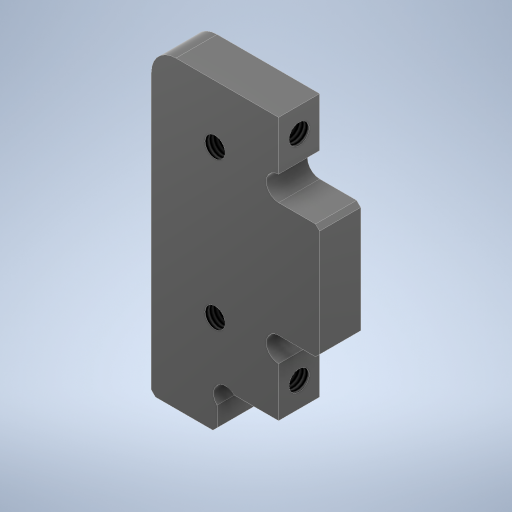
# Autodesk Inventor part: TorsoAngleBraceFrame
Saved by Autodesk Inventor 2024.2 (Build 282272000, 272)
## iProperties
Created: 2024-01-21
Part Number: TorsoAngleBraceFrame
Material: Acetal Resin, Black
Document SubType Name: Modeling
Designer: Masato Kubotera
Density: 1.425 g/cm^3
Appearance: Smooth - Black
Mass: 4.09203 g
Surface Area: 19.2357 cm^2
Volume: 2.8716 cm^3
Vendor: meviy
Author: Masato Kubotera
Autodesk Inventor part; units mm, degrees
ref_plane "YZ Plane" through (0, 0, 0) normal (1, 0, 0) x (0, 1, 0)
ref_plane "XZ Plane" through (0, 0, 0) normal (0, 1, 0) x (-1, 0, 0)
ref_plane "XY Plane" through (0, 0, 0) normal (0, 0, 1) x (1, 0, 0)
sketch "Sketch1" plane through (0, 0, 0) normal (1, 0, 0) x (0, 1, 0)
  line L0 (0.25, 0) -> (0.25, -5)
  line L1 (0.25, -5) -> (-7.75, -5)
  line L2 (-7.75, -5) -> (-7.75, 32)
  line L3 (-7.75, 32) -> (7.75, 32)
  line L4 (7.75, 32) -> (7.75, 23)
  line L5 (7.75, 23) -> (12.75, 23)
  line L6 (12.75, 23) -> (12.75, 9)
  line L7 (12.75, 9) -> (7.75, 9)
  line L8 (0.25, 0) -> (7.75, 0)
  line L9 (7.75, 0) -> (7.75, 9)
  line L10 (0, -5) -> (0, 32) construction
  line L11 (12.75, 16) -> (-7.75, 16) construction
  arc A0 (7.75, 26) -> (7.75, 23) centre (7.75, 24.5) ccw
  arc A1 (7.75, 9) -> (7.75, 6) centre (7.75, 7.5) ccw
  arc A2 (2.3713, 0) -> (0.25, -2.1213) centre (1.3107, -1.0607) ccw
  line L12 (7.75, 29) -> (1.75, 29) construction
  line L13 (7.75, 3) -> (1.75, 3) construction
  point P0 (0, 0)
  point P1 (0, 25)
  point P2 (0, 7)
  point P3 (7.75, 6)
  point P4 (4.1709, -1.359)
  point P5 (4.291, 0)
  dimension "d6" = 5
  dimension "d7" = 14
  dimension "d8" = 5
  dimension "d9" = 18
  dimension "d12" = 6
  dimension "d13" = 6
  dimension "d31" = 9
  dimension "d32" = 1.5
  dimension "d33" = 32
  dimension "d34" = 8
  dimension "d35" = 15.5
  constraints: 28 end point, 11 point on line, 7 horizontal, 7 point on circle, 6 vertical, 5 symmetric about line, 3 centre point, 2 midpoint, 1 equal radius, 3 other
  measures "d6" distance of L0.start L0.end
  measures "d7" distance of L5.end L6.end
  measures "d8" distance of L6.end L7.end
  measures "d9" distance of point (0, 7) point (0, 25)
  measures "d12" distance of L12.start L12.end
  measures "d13" diameter of L3 L12
  measures "d31" distance between parallel lines of L5 L3
  measures "d32" radius of A2
  measures "d33" distance between parallel lines of L8 L3
  measures "d34" distance of L0.end L1.end
  measures "d35" distance of L2.end L3.end
extrude "Extrusion1" add sketch "Sketch1" along normal blind 5 contours A2 L0 L1 L2 L3 L4 A0 L5 L6 L7 A1 L9 L8
sketch "Sketch2" plane through (0, 7.75, 32) normal (0, 1, 0) x (1, 0, 0)
  line L0 (5, 3) -> (0, 3)
  line L1 (0, 9) -> (0, 0) projected
  line L2 (5, 32) -> (5, 23) projected
  line L3 (5, 29) -> (0, 29)
  line L4 (5, 9) -> (5, 0) projected
  point P0 (0, 32)
  point P1 (0, 6)
  point P2 (5, 26)
  point P3 (5, 6)
  point P4 (0, 29)
  point P5 (0, 29)
  point P6 (0, 29)
  point P7 (2.5, 29)
  point P8 (2.5, 3)
  constraints: 4 end point, 2 horizontal, 2 midpoint, 2 point on line, 1 coincident
hole "Hole1" at (2.5, 7.75, 3) at (2.5, 7.75, 29) direction (0, -1, 0) diameter 2.459 depth 6 thread size "M3x0.5" class "6H" standard "ANSI Metric M Profile"
hole "Hole2" at (0, 0, 25) at (0, 0, 7) direction (1, 0, 0) diameter 2.459 end through all thread size "M3x0.5" class "6H" standard "ANSI Metric M Profile"
chamfer "Chamfer1" distance 0.5 angle 45 4 edges at (2.5, -7.75, -5) (2.5, 0.25, -5) (2.5, 12.75, 9) (2.5, 12.75, 23)
fillet "Fillet1" radius 3 1 edges at (2.5, -7.75, 32)
body "Solid1"
